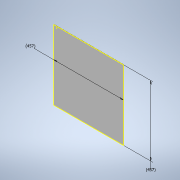
# Autodesk Inventor part: upperplate01
Saved by Autodesk Inventor 2021 (Build 250183000, 183)
## iProperties
Created: 2023-06-07
Part Number: upperplate01
Material: Generic
Document SubType Name: Modeling
Designer: badig
Density: 1 g/cm^3
Appearance: Default
Author: badig
Autodesk Inventor part; units mm, degrees
ref_plane "YZ Plane" through (0, 0, 0) normal (1, 0, 0) x (0, 1, 0)
ref_plane "XZ Plane" through (0, 0, 0) normal (0, 1, 0) x (-1, 0, 0)
ref_plane "XY Plane" through (0, 0, 0) normal (0, 0, 1) x (1, 0, 0)
sketch "Sketch1" plane through (0, 0, 0) normal (0, 0, 1) x (1, 0, 0)
  line L0 (-18.7595, 10.7292) -> (438.2405, 10.7292)
  line L1 (438.2405, 10.7292) -> (438.2405, -446.2708)
  line L2 (438.2405, -446.2708) -> (-18.7595, -446.2708)
  line L3 (-18.7595, -446.2708) -> (-18.7595, 10.7292)
  point P0 (0, 0)
  dimension "d0" = 457
  dimension "d1" = 457
  constraints: 8 end point, 2 parallel, 1 horizontal, 1 perpendicular
  measures "d0" distance of L1.end L2.end
  measures "d1" distance of L0.end L1.end
extrude "Extrusion1" add sketch "Sketch1" along normal blind 2
sketch "Sketch2" plane through (0, 0, 2) normal (0, 0, 1) x (1, 0, 0)
  line L0 (-18.7595, 10.7292) -> (-18.7595, -446.2708) projected
  line L1 (438.2405, -446.2708) -> (438.2405, 10.7292) projected
  line L2 (-18.7595, -446.2708) -> (438.2405, -446.2708) projected
  line L3 (438.2405, 10.7292) -> (-18.7595, 10.7292) projected
  point P0 (0, 0)
  dimension "d4" = 457
  dimension "d5" = 457
  measures "d4" distance between parallel lines of L0 L1
  measures "d5" distance between parallel lines of L2 L3
body "Solid1"
